Autodesk Inventor part; units mm, degrees
(part 2 of 3)
  arc A433 (-195.284, 57.8625) -> (-192.1375, 54.716) centre (-190, 60) ccw construction
  arc A434 (-198.1598, 81.4621) -> (-195.284, 57.8625) centre (-152.919, 75) ccw construction
  arc A435 (-196.5476, 84.6866) -> (-198.1598, 81.4621) centre (-192.5171, 80.6561) ccw construction
  line L149 (-196.5476, 84.6866) -> (-178.0824, 103.1518) construction
  arc A436 (-171.9305, 105.7) -> (-178.0824, 103.1518) centre (-171.9305, 97) ccw construction
  line L150 (-171.9305, 105.7) -> (-161.9122, 105.7) construction
  arc A437 (-192.1375, 45.284) -> (-195.284, 42.1375) centre (-190, 40) ccw construction
  arc A438 (-157.8625, 45.284) -> (-192.1375, 45.284) centre (-175, 2.919) ccw construction
  arc A439 (-154.716, 42.1375) -> (-157.8625, 45.284) centre (-160, 40) ccw construction
  arc A440 (-154.716, 7.8625) -> (-154.716, 42.1375) centre (-197.081, 25) ccw construction
  arc A441 (-157.8625, 4.716) -> (-154.716, 7.8625) centre (-160, 10) ccw construction
  arc A442 (-192.1375, 4.716) -> (-157.8625, 4.716) centre (-175, 47.081) ccw construction
  arc A443 (-195.284, 7.8625) -> (-192.1375, 4.716) centre (-190, 10) ccw construction
  arc A444 (-195.284, 42.1375) -> (-195.284, 7.8625) centre (-152.919, 25) ccw construction
  arc A445 (-192.1375, -4.716) -> (-195.284, -7.8625) centre (-190, -10) ccw construction
  arc A446 (-157.8625, -4.716) -> (-192.1375, -4.716) centre (-175, -47.081) ccw construction
  arc A447 (-154.716, -7.8625) -> (-157.8625, -4.716) centre (-160, -10) ccw construction
  arc A448 (-154.716, -42.1375) -> (-154.716, -7.8625) centre (-197.081, -25) ccw construction
  arc A449 (-157.8625, -45.284) -> (-154.716, -42.1375) centre (-160, -40) ccw construction
  arc A450 (-192.1375, -45.284) -> (-157.8625, -45.284) centre (-175, -2.919) ccw construction
  arc A451 (-195.284, -42.1375) -> (-192.1375, -45.284) centre (-190, -40) ccw construction
  arc A452 (-195.284, -7.8625) -> (-195.284, -42.1375) centre (-152.919, -25) ccw construction
  line L151 (-172.8179, -78.4527) -> (-172.8179, -89.3404) construction
  arc A453 (-183.0505, -97.9043) -> (-172.8179, -89.3404) centre (-181.5179, -89.3404) ccw construction
  arc A454 (-192.1375, -95.284) -> (-183.0505, -97.9043) centre (-175, -52.919) ccw construction
  arc A455 (-195.284, -92.1375) -> (-192.1375, -95.284) centre (-190, -90) ccw construction
  arc A456 (-195.284, -57.8625) -> (-195.284, -92.1375) centre (-152.919, -75) ccw construction
  arc A457 (-192.1375, -54.716) -> (-195.284, -57.8625) centre (-190, -60) ccw construction
  arc A458 (-171.3004, -51.531) -> (-192.1375, -54.716) centre (-175, -97.081) ccw construction
  arc A459 (-164.8787, -65.1933) -> (-171.3004, -51.531) centre (-172.0047, -60.2024) ccw construction
  line L152 (-164.8787, -65.1933) -> (-171.7143, -74.9534) construction
  arc A460 (-171.7143, -74.9534) -> (-172.8179, -78.4527) centre (-166.7179, -78.4527) ccw construction
  arc A461 (-195.284, -107.8625) -> (-198.5651, -122.7803) centre (-152.919, -125) ccw construction
  arc A462 (-192.1375, -104.716) -> (-195.284, -107.8625) centre (-190, -110) ccw construction
  arc A463 (-168.9997, -101.7766) -> (-192.1375, -104.716) centre (-175, -147.081) ccw construction
  arc A464 (-163.9859, -111.6056) -> (-168.9997, -101.7766) centre (-169.8794, -108.4186) ccw construction
  arc A465 (-163.9859, -111.6056) -> (-158.7814, -119.3988) centre (-159.3239, -114.1267) ccw construction
  arc A466 (-151.398, -126.2464) -> (-158.7814, -119.3988) centre (-158.0955, -126.0637) ccw construction
  arc A467 (-154.716, -142.1375) -> (-151.398, -126.2464) centre (-197.081, -125) ccw construction
  arc A468 (-157.8625, -145.284) -> (-154.716, -142.1375) centre (-160, -140) ccw construction
  arc A469 (-181.1757, -148.1998) -> (-157.8625, -145.284) centre (-175, -102.919) ccw construction
  arc A470 (-188.7, -139.5796) -> (-181.1757, -148.1998) centre (-180, -139.5796) ccw construction
  line L153 (-188.7, -139.5796) -> (-188.7, -137.0711) construction
  arc A471 (-188.7, -137.0711) -> (-189.9594, -134.0305) centre (-193, -137.0711) ccw construction
  line L154 (-189.9594, -134.0305) -> (-196.9023, -127.0876) construction
  arc A472 (-198.5651, -122.7803) -> (-196.9023, -127.0876) centre (-192.8718, -123.0571) ccw construction
  arc A473 (-157.8625, -154.716) -> (-171.7212, -151.4988) centre (-175, -197.081) ccw construction
  arc A474 (-154.716, -157.8625) -> (-157.8625, -154.716) centre (-160, -160) ccw construction
  arc A475 (-151.4988, -171.7212) -> (-154.716, -157.8625) centre (-197.081, -175) ccw construction
  arc A476 (-166.4392, -178.3841) -> (-151.4988, -171.7212) centre (-160.1763, -172.3454) ccw construction
  arc A477 (-166.4392, -178.3841) -> (-178.3841, -166.4392) centre (-500.278, -500.278) ccw construction
  arc A478 (-171.7212, -151.4988) -> (-178.3841, -166.4392) centre (-172.3454, -160.1763) ccw construction
  arc A479 (-107.8625, -195.284) -> (-104.716, -192.1375) centre (-110, -190) ccw construction
  arc A480 (-142.1375, -195.284) -> (-107.8625, -195.284) centre (-125, -152.919) ccw construction
  arc A481 (-145.284, -192.1375) -> (-142.1375, -195.284) centre (-140, -190) ccw construction
  arc A482 (-145.284, -157.8625) -> (-145.284, -192.1375) centre (-102.919, -175) ccw construction
  arc A483 (-142.1375, -154.716) -> (-145.284, -157.8625) centre (-140, -160) ccw construction
  arc A484 (-107.8625, -154.716) -> (-142.1375, -154.716) centre (-125, -197.081) ccw construction
  arc A485 (-104.716, -157.8625) -> (-107.8625, -154.716) centre (-110, -160) ccw construction
  arc A486 (-104.716, -192.1375) -> (-104.716, -157.8625) centre (-147.081, -175) ccw construction
  arc A487 (-128.4924, -148.4854) -> (-107.8625, -145.284) centre (-125, -102.919) ccw construction
  arc A488 (-133.4107, -144.758) -> (-128.4924, -148.4854) centre (-128.0568, -142.802) ccw construction
  arc A489 (-133.4107, -144.758) -> (-139.1817, -140.7513) centre (-139.1403, -146.8512) ccw construction
  arc A490 (-147.7814, -133.7096) -> (-139.1817, -140.7513) centre (-139.2409, -132.0515) ccw construction
  arc A491 (-145.284, -107.8625) -> (-147.7814, -133.7096) centre (-102.919, -125) ccw construction
  arc A492 (-142.1375, -104.716) -> (-145.284, -107.8625) centre (-140, -110) ccw construction
  arc A493 (-107.8625, -104.716) -> (-142.1375, -104.716) centre (-125, -147.081) ccw construction
  arc A494 (-104.716, -107.8625) -> (-107.8625, -104.716) centre (-110, -110) ccw construction
  arc A495 (-104.716, -142.1375) -> (-104.716, -107.8625) centre (-147.081, -125) ccw construction
  arc A496 (-107.8625, -145.284) -> (-104.716, -142.1375) centre (-110, -140) ccw construction
  arc A497 (-139.6902, -96.1936) -> (-142.6797, -95.7) centre (-142.6797, -105) ccw construction
  line L155 (-142.6797, -95.7) -> (-156, -95.7) construction
  arc A498 (-160.7, -91) -> (-156, -95.7) centre (-156, -91) ccw construction
  line L156 (-160.7, -91) -> (-160.7, -82.9939) construction
  arc A499 (-158.7642, -76.8556) -> (-160.7, -82.9939) centre (-150, -82.9939) ccw construction
  line L157 (-158.7642, -76.8556) -> (-144.6688, -56.7301) construction
  arc A500 (-142.1375, -54.716) -> (-144.6688, -56.7301) centre (-140, -60) ccw construction
  arc A501 (-107.8625, -54.716) -> (-142.1375, -54.716) centre (-125, -97.081) ccw construction
  arc A502 (-104.716, -57.8625) -> (-107.8625, -54.716) centre (-110, -60) ccw construction
  arc A503 (-104.716, -92.1375) -> (-104.716, -57.8625) centre (-147.081, -75) ccw construction
  arc A504 (-107.8625, -95.284) -> (-104.716, -92.1375) centre (-110, -90) ccw construction
  arc A505 (-139.6902, -96.1936) -> (-107.8625, -95.284) centre (-125, -52.919) ccw construction
  arc A506 (-142.1375, -4.716) -> (-145.284, -7.8625) centre (-140, -10) ccw construction
  arc A507 (-107.8625, -4.716) -> (-142.1375, -4.716) centre (-125, -47.081) ccw construction
  arc A508 (-104.716, -7.8625) -> (-107.8625, -4.716) centre (-110, -10) ccw construction
  arc A509 (-104.716, -42.1375) -> (-104.716, -7.8625) centre (-147.081, -25) ccw construction
  arc A510 (-107.8625, -45.284) -> (-104.716, -42.1375) centre (-110, -40) ccw construction
  arc A511 (-142.1375, -45.284) -> (-107.8625, -45.284) centre (-125, -2.919) ccw construction
  arc A512 (-145.284, -42.1375) -> (-142.1375, -45.284) centre (-140, -40) ccw construction
  arc A513 (-145.284, -7.8625) -> (-145.284, -42.1375) centre (-102.919, -25) ccw construction
  arc A514 (-92.1375, 45.284) -> (-95.284, 42.1375) centre (-90, 40) ccw construction
  arc A515 (-57.8625, 45.284) -> (-92.1375, 45.284) centre (-75, 2.919) ccw construction
  arc A516 (-54.716, 42.1375) -> (-57.8625, 45.284) centre (-60, 40) ccw projected
  arc A517 (-54.716, 7.8625) -> (-54.716, 42.1375) centre (-97.081, 25) ccw projected
  arc A518 (-57.8625, 4.716) -> (-54.716, 7.8625) centre (-60, 10) ccw projected
  arc A519 (-92.1375, 4.716) -> (-57.8625, 4.716) centre (-75, 47.081) ccw construction
  arc A520 (-95.284, 7.8625) -> (-92.1375, 4.716) centre (-90, 10) ccw construction
  arc A521 (-95.284, 42.1375) -> (-95.284, 7.8625) centre (-52.919, 25) ccw construction
  arc A522 (-45.3096, 30.6473) -> (-44.8166, 8.2343) centre (-7.9112, 20.258) ccw projected
  arc A523 (-29.5673, 37.0015) -> (-45.3096, 30.6473) centre (-35, 27.7833) ccw projected
  arc A524 (-29.5673, 37.0015) -> (-20.8305, 37.1926) centre (-25.3532, 44.1521) ccw projected
  arc A525 (-5.5366, 33.2142) -> (-20.8305, 37.1926) centre (-15, 28.2207) ccw projected
  arc A526 (-8.2916, 26.5347) -> (-5.5366, 33.2142) centre (-9.6934, 31.0208) ccw projected
  arc A527 (-8.2916, 26.5347) -> (-26.7128, 7.6985) centre (0, 0) ccw projected
  arc A528 (-31.229, 4.3) -> (-26.7128, 7.6985) centre (-31.229, 9) ccw projected
  line L158 (-31.229, 4.3) -> (-39.3969, 4.3) projected
  arc A529 (-44.8166, 8.2343) -> (-39.3969, 4.3) centre (-39.3969, 10) ccw projected
  arc A530 (-30.6473, -45.3096) -> (-8.2343, -44.8166) centre (-20.258, -7.9112) ccw projected
  arc A531 (-37.0015, -29.5673) -> (-30.6473, -45.3096) centre (-27.7833, -35) ccw projected
  arc A532 (-37.0015, -29.5673) -> (-37.1926, -20.8305) centre (-44.1521, -25.3532) ccw projected
  arc A533 (-33.2142, -5.5366) -> (-37.1926, -20.8305) centre (-28.2207, -15) ccw projected
  arc A534 (-26.5347, -8.2916) -> (-33.2142, -5.5366) centre (-31.0208, -9.6934) ccw projected
  arc A535 (-26.5347, -8.2916) -> (-7.6985, -26.7128) centre (0, 0) ccw projected
  arc A536 (-4.3, -31.229) -> (-7.6985, -26.7128) centre (-9, -31.229) ccw projected
  line L159 (-4.3, -31.229) -> (-4.3, -39.3969) projected
  arc A537 (-8.2343, -44.8166) -> (-4.3, -39.3969) centre (-10, -39.3969) ccw projected
  arc A538 (-92.1375, -4.716) -> (-95.284, -7.8625) centre (-90, -10) ccw construction
  arc A539 (-57.8625, -4.716) -> (-92.1375, -4.716) centre (-75, -47.081) ccw construction
  arc A540 (-54.716, -7.8625) -> (-57.8625, -4.716) centre (-60, -10) ccw projected
  arc A541 (-54.716, -42.1375) -> (-54.716, -7.8625) centre (-97.081, -25) ccw projected
  arc A542 (-57.8625, -45.284) -> (-54.716, -42.1375) centre (-60, -40) ccw projected
  arc A543 (-92.1375, -45.284) -> (-57.8625, -45.284) centre (-75, -2.919) ccw construction
  arc A544 (-95.284, -42.1375) -> (-92.1375, -45.284) centre (-90, -40) ccw construction
  arc A545 (-95.284, -7.8625) -> (-95.284, -42.1375) centre (-52.919, -25) ccw construction
  arc A546 (-92.1375, -54.716) -> (-95.284, -57.8625) centre (-90, -60) ccw construction
  arc A547 (-57.8625, -54.716) -> (-92.1375, -54.716) centre (-75, -97.081) ccw construction
  arc A548 (-54.716, -57.8625) -> (-57.8625, -54.716) centre (-60, -60) ccw projected
  arc A549 (-54.716, -92.1375) -> (-54.716, -57.8625) centre (-97.081, -75) ccw construction
  arc A550 (-57.8625, -95.284) -> (-54.716, -92.1375) centre (-60, -90) ccw construction
  arc A551 (-92.1375, -95.284) -> (-57.8625, -95.284) centre (-75, -52.919) ccw construction
  arc A552 (-95.284, -92.1375) -> (-92.1375, -95.284) centre (-90, -90) ccw construction
  arc A553 (-95.284, -57.8625) -> (-95.284, -92.1375) centre (-52.919, -75) ccw construction
  arc A554 (-92.1375, -104.716) -> (-95.284, -107.8625) centre (-90, -110) ccw construction
  arc A555 (-57.8625, -104.716) -> (-92.1375, -104.716) centre (-75, -147.081) ccw construction
  arc A556 (-54.716, -107.8625) -> (-57.8625, -104.716) centre (-60, -110) ccw construction
  arc A557 (-54.716, -142.1375) -> (-54.716, -107.8625) centre (-97.081, -125) ccw construction
  arc A558 (-57.8625, -145.284) -> (-54.716, -142.1375) centre (-60, -140) ccw construction
  arc A559 (-92.1375, -145.284) -> (-57.8625, -145.284) centre (-75, -102.919) ccw construction
  arc A560 (-95.284, -142.1375) -> (-92.1375, -145.284) centre (-90, -140) ccw construction
  arc A561 (-95.284, -107.8625) -> (-95.284, -142.1375) centre (-52.919, -125) ccw construction
  arc A562 (-92.1375, -154.716) -> (-95.284, -157.8625) centre (-90, -160) ccw construction
  arc A563 (-57.8625, -154.716) -> (-92.1375, -154.716) centre (-75, -197.081) ccw construction
  arc A564 (-54.716, -157.8625) -> (-57.8625, -154.716) centre (-60, -160) ccw construction
  arc A565 (-54.716, -192.1375) -> (-54.716, -157.8625) centre (-97.081, -175) ccw construction
  arc A566 (-57.8625, -195.284) -> (-54.716, -192.1375) centre (-60, -190) ccw construction
  arc A567 (-92.1375, -195.284) -> (-57.8625, -195.284) centre (-75, -152.919) ccw construction
  arc A568 (-95.284, -192.1375) -> (-92.1375, -195.284) centre (-90, -190) ccw construction
  arc A569 (-95.284, -157.8625) -> (-95.284, -192.1375) centre (-52.919, -175) ccw construction
  arc A570 (30.6473, 45.3096) -> (8.2343, 44.8166) centre (20.258, 7.9112) ccw projected
  arc A571 (37.0015, 29.5673) -> (30.6473, 45.3096) centre (27.7833, 35) ccw projected
  arc A572 (37.0015, 29.5673) -> (37.1926, 20.8305) centre (44.1521, 25.3532) ccw projected
  arc A573 (33.2142, 5.5366) -> (37.1926, 20.8305) centre (28.2207, 15) ccw projected
  arc A574 (26.5347, 8.2916) -> (33.2142, 5.5366) centre (31.0208, 9.6934) ccw projected
  arc A575 (26.5347, 8.2916) -> (7.6985, 26.7128) centre (0, 0) ccw projected
  arc A576 (4.3, 31.229) -> (7.6985, 26.7128) centre (9, 31.229) ccw projected
  line L160 (4.3, 31.229) -> (4.3, 39.3969) projected
  arc A577 (8.2343, 44.8166) -> (4.3, 39.3969) centre (10, 39.3969) ccw projected
  arc A578 (8.2916, -26.5347) -> (5.5366, -33.2142) centre (9.6934, -31.0208) ccw projected
  arc A579 (8.2916, -26.5347) -> (26.7128, -7.6985) centre (0, 0) ccw projected
  arc A580 (31.229, -4.3) -> (26.7128, -7.6985) centre (31.229, -9) ccw projected
  line L161 (31.229, -4.3) -> (39.3969, -4.3) projected
  arc A581 (44.8166, -8.2343) -> (39.3969, -4.3) centre (39.3969, -10) ccw projected
  arc A582 (45.3096, -30.6473) -> (44.8166, -8.2343) centre (7.9112, -20.258) ccw projected
  arc A583 (29.5673, -37.0015) -> (45.3096, -30.6473) centre (35, -27.7833) ccw projected
  arc A584 (29.5673, -37.0015) -> (20.8305, -37.1926) centre (25.3532, -44.1521) ccw projected
  arc A585 (5.5366, -33.2142) -> (20.8305, -37.1926) centre (15, -28.2207) ccw projected
  arc A586 (57.8625, 45.284) -> (54.716, 42.1375) centre (60, 40) ccw projected
  arc A587 (92.1375, 45.284) -> (57.8625, 45.284) centre (75, 2.919) ccw construction
  arc A588 (95.284, 42.1375) -> (92.1375, 45.284) centre (90, 40) ccw construction
  arc A589 (95.284, 7.8625) -> (95.284, 42.1375) centre (52.919, 25) ccw construction
  arc A590 (92.1375, 4.716) -> (95.284, 7.8625) centre (90, 10) ccw construction
  arc A591 (57.8625, 4.716) -> (92.1375, 4.716) centre (75, 47.081) ccw construction
  arc A592 (54.716, 7.8625) -> (57.8625, 4.716) centre (60, 10) ccw projected
  arc A593 (54.716, 42.1375) -> (54.716, 7.8625) centre (97.081, 25) ccw projected
  arc A594 (57.8625, -4.716) -> (54.716, -7.8625) centre (60, -10) ccw projected
  arc A595 (92.1375, -4.716) -> (57.8625, -4.716) centre (75, -47.081) ccw construction
  arc A596 (95.284, -7.8625) -> (92.1375, -4.716) centre (90, -10) ccw construction
  arc A597 (95.284, -42.1375) -> (95.284, -7.8625) centre (52.919, -25) ccw construction
  arc A598 (92.1375, -45.284) -> (95.284, -42.1375) centre (90, -40) ccw construction
  arc A599 (57.8625, -45.284) -> (92.1375, -45.284) centre (75, -2.919) ccw construction
  arc A600 (54.716, -42.1375) -> (57.8625, -45.284) centre (60, -40) ccw projected
  arc A601 (54.716, -7.8625) -> (54.716, -42.1375) centre (97.081, -25) ccw projected
  arc A602 (157.8625, 45.284) -> (154.716, 42.1375) centre (160, 40) ccw construction
  arc A603 (192.1375, 45.284) -> (157.8625, 45.284) centre (175, 2.919) ccw construction
  arc A604 (195.284, 42.1375) -> (192.1375, 45.284) centre (190, 40) ccw construction
  arc A605 (195.284, 7.8625) -> (195.284, 42.1375) centre (152.919, 25) ccw construction
  arc A606 (192.1375, 4.716) -> (195.284, 7.8625) centre (190, 10) ccw construction
  arc A607 (157.8625, 4.716) -> (192.1375, 4.716) centre (175, 47.081) ccw construction
  arc A608 (154.716, 7.8625) -> (157.8625, 4.716) centre (160, 10) ccw construction
  arc A609 (154.716, 42.1375) -> (154.716, 7.8625) centre (197.081, 25) ccw construction
  arc A610 (107.8625, 45.284) -> (104.716, 42.1375) centre (110, 40) ccw construction
  arc A611 (142.1375, 45.284) -> (107.8625, 45.284) centre (125, 2.919) ccw construction
  arc A612 (145.284, 42.1375) -> (142.1375, 45.284) centre (140, 40) ccw construction
  arc A613 (145.284, 7.8625) -> (145.284, 42.1375) centre (102.919, 25) ccw construction
  arc A614 (142.1375, 4.716) -> (145.284, 7.8625) centre (140, 10) ccw construction
  arc A615 (107.8625, 4.716) -> (142.1375, 4.716) centre (125, 47.081) ccw construction
  arc A616 (104.716, 7.8625) -> (107.8625, 4.716) centre (110, 10) ccw construction
  arc A617 (104.716, 42.1375) -> (104.716, 7.8625) centre (147.081, 25) ccw construction
  arc A618 (107.8625, -4.716) -> (104.716, -7.8625) centre (110, -10) ccw construction
  arc A619 (142.1375, -4.716) -> (107.8625, -4.716) centre (125, -47.081) ccw construction
  arc A620 (145.284, -7.8625) -> (142.1375, -4.716) centre (140, -10) ccw construction
  arc A621 (145.284, -42.1375) -> (145.284, -7.8625) centre (102.919, -25) ccw construction
  arc A622 (142.1375, -45.284) -> (145.284, -42.1375) centre (140, -40) ccw construction
  arc A623 (107.8625, -45.284) -> (142.1375, -45.284) centre (125, -2.919) ccw construction
  arc A624 (104.716, -42.1375) -> (107.8625, -45.284) centre (110, -40) ccw construction
  arc A625 (104.716, -7.8625) -> (104.716, -42.1375) centre (147.081, -25) ccw construction
  arc A626 (157.8625, -4.716) -> (154.716, -7.8625) centre (160, -10) ccw construction
  arc A627 (192.1375, -4.716) -> (157.8625, -4.716) centre (175, -47.081) ccw construction
  arc A628 (195.284, -7.8625) -> (192.1375, -4.716) centre (190, -10) ccw construction
  arc A629 (195.284, -42.1375) -> (195.284, -7.8625) centre (152.919, -25) ccw construction
  arc A630 (192.1375, -45.284) -> (195.284, -42.1375) centre (190, -40) ccw construction
  arc A631 (157.8625, -45.284) -> (192.1375, -45.284) centre (175, -2.919) ccw construction
  arc A632 (154.716, -42.1375) -> (157.8625, -45.284) centre (160, -40) ccw construction
  arc A633 (154.716, -7.8625) -> (154.716, -42.1375) centre (197.081, -25) ccw construction
  line L162 (157.3723, -102.2164) -> (154.5817, -91.8019) construction
  arc A634 (154.716, -57.8625) -> (154.5817, -91.8019) centre (197.081, -75) ccw construction
  arc A635 (157.8625, -54.716) -> (154.716, -57.8625) centre (160, -60) ccw construction
  arc A636 (192.1375, -54.716) -> (157.8625, -54.716) centre (175, -97.081) ccw construction
  arc A637 (195.284, -57.8625) -> (192.1375, -54.716) centre (190, -60) ccw construction
  arc A638 (198.1598, -81.4621) -> (195.284, -57.8625) centre (152.919, -75) ccw construction
  arc A639 (196.5476, -84.6866) -> (198.1598, -81.4621) centre (192.5171, -80.6561) ccw construction
  line L163 (196.5476, -84.6866) -> (178.0824, -103.1518) construction
  arc A640 (171.9305, -105.7) -> (178.0824, -103.1518) centre (171.9305, -97) ccw construction
  line L164 (171.9305, -105.7) -> (161.9122, -105.7) construction
  arc A641 (157.3723, -102.2164) -> (161.9122, -105.7) centre (161.9122, -101) ccw construction
  arc A642 (188.629, -104.3) -> (184.5985, -105.9695) centre (188.629, -110) ccw construction
  line L165 (188.629, -104.3) -> (190, -104.3) construction
  arc A643 (195.284, -107.8625) -> (190, -104.3) centre (190, -110) ccw construction
  arc A644 (198.5651, -122.7803) -> (195.284, -107.8625) centre (152.919, -125) ccw construction
  arc A645 (196.9023, -127.0876) -> (198.5651, -122.7803) centre (192.8718, -123.0571) ccw construction
  line L166 (196.9023, -127.0876) -> (189.9594, -134.0305) construction
  arc A646 (189.9594, -134.0305) -> (188.7, -137.0711) centre (193, -137.0711) ccw construction
  line L167 (188.7, -137.0711) -> (188.7, -139.5796) construction
  arc A647 (181.1757, -148.1998) -> (188.7, -139.5796) centre (180, -139.5796) ccw construction
  arc A648 (157.8625, -145.284) -> (181.1757, -148.1998) centre (175, -102.919) ccw construction
  arc A649 (154.716, -142.1375) -> (157.8625, -145.284) centre (160, -140) ccw construction
  arc A650 (151.6379, -129.8385) -> (154.716, -142.1375) centre (197.081, -125) ccw construction
  arc A651 (160.289, -120.2174) -> (151.6379, -129.8385) centre (160.289, -128.9174) ccw construction
  line L168 (160.289, -120.2174) -> (167.8239, -120.2174) construction
  arc A652 (167.8239, -120.2174) -> (172.1372, -118.4308) centre (167.8239, -114.1174) ccw construction
  line L169 (172.1372, -118.4308) -> (184.5985, -105.9695) construction
  arc A653 (195.3029, -159.9476) -> (191.4845, -156.1292) centre (193.3937, -158.0384) ccw construction
  line L170 (195.3029, -159.9476) -> (159.9476, -195.3029) construction
  arc A654 (156.1292, -191.4845) -> (159.9476, -195.3029) centre (158.0384, -193.3937) ccw construction
  line L171 (156.1292, -191.4845) -> (191.4845, -156.1292) construction
  arc A655 (154.716, -157.8625) -> (151.4988, -171.7212) centre (197.081, -175) ccw construction
  arc A656 (157.8625, -154.716) -> (154.716, -157.8625) centre (160, -160) ccw construction
  arc A657 (171.7212, -151.4988) -> (157.8625, -154.716) centre (175, -197.081) ccw construction
  arc A658 (178.3841, -166.4392) -> (171.7212, -151.4988) centre (172.3454, -160.1763) ccw construction
  arc A659 (178.3841, -166.4392) -> (166.4392, -178.3841) centre (500.278, -500.278) ccw construction
  arc A660 (151.4988, -171.7212) -> (166.4392, -178.3841) centre (160.1763, -172.3454) ccw construction
  arc A661 (-42.1375, -54.716) -> (-45.284, -57.8625) centre (-40, -60) ccw projected
  arc A662 (-7.8625, -54.716) -> (-42.1375, -54.716) centre (-25, -97.081) ccw projected
  arc A663 (-4.716, -57.8625) -> (-7.8625, -54.716) centre (-10, -60) ccw projected
  arc A664 (-4.716, -92.1375) -> (-4.716, -57.8625) centre (-47.081, -75) ccw construction
  arc A665 (-7.8625, -95.284) -> (-4.716, -92.1375) centre (-10, -90) ccw construction
  arc A666 (-42.1375, -95.284) -> (-7.8625, -95.284) centre (-25, -52.919) ccw construction
  arc A667 (-45.284, -92.1375) -> (-42.1375, -95.284) centre (-40, -90) ccw construction
  arc A668 (-45.284, -57.8625) -> (-45.284, -92.1375) centre (-2.919, -75) ccw construction
  arc A669 (7.8625, -54.716) -> (4.716, -57.8625) centre (10, -60) ccw projected
  arc A670 (42.1375, -54.716) -> (7.8625, -54.716) centre (25, -97.081) ccw projected
  arc A671 (45.284, -57.8625) -> (42.1375, -54.716) centre (40, -60) ccw projected
  arc A672 (45.284, -92.1375) -> (45.284, -57.8625) centre (2.919, -75) ccw construction
  arc A673 (42.1375, -95.284) -> (45.284, -92.1375) centre (40, -90) ccw construction
  arc A674 (7.8625, -95.284) -> (42.1375, -95.284) centre (25, -52.919) ccw construction
  arc A675 (4.716, -92.1375) -> (7.8625, -95.284) centre (10, -90) ccw construction
  arc A676 (4.716, -57.8625) -> (4.716, -92.1375) centre (47.081, -75) ccw construction
  arc A677 (57.8625, -54.716) -> (54.716, -57.8625) centre (60, -60) ccw projected
  arc A678 (92.1375, -54.716) -> (57.8625, -54.716) centre (75, -97.081) ccw construction
  arc A679 (95.284, -57.8625) -> (92.1375, -54.716) centre (90, -60) ccw construction
  arc A680 (95.284, -92.1375) -> (95.284, -57.8625) centre (52.919, -75) ccw construction
  arc A681 (92.1375, -95.284) -> (95.284, -92.1375) centre (90, -90) ccw construction
  arc A682 (57.8625, -95.284) -> (92.1375, -95.284) centre (75, -52.919) ccw construction
  arc A683 (54.716, -92.1375) -> (57.8625, -95.284) centre (60, -90) ccw construction
  arc A684 (54.716, -57.8625) -> (54.716, -92.1375) centre (97.081, -75) ccw construction
  arc A685 (107.8625, -54.716) -> (104.716, -57.8625) centre (110, -60) ccw construction
  arc A686 (142.1375, -54.716) -> (107.8625, -54.716) centre (125, -97.081) ccw construction
  arc A687 (145.284, -57.8625) -> (142.1375, -54.716) centre (140, -60) ccw construction
  arc A688 (145.284, -92.1375) -> (145.284, -57.8625) centre (102.919, -75) ccw construction
  arc A689 (142.1375, -95.284) -> (145.284, -92.1375) centre (140, -90) ccw construction
  arc A690 (107.8625, -95.284) -> (142.1375, -95.284) centre (125, -52.919) ccw construction
  arc A691 (104.716, -92.1375) -> (107.8625, -95.284) centre (110, -90) ccw construction
  arc A692 (104.716, -57.8625) -> (104.716, -92.1375) centre (147.081, -75) ccw construction
  arc A693 (107.8625, -104.716) -> (104.716, -107.8625) centre (110, -110) ccw construction
  arc A694 (142.1375, -104.716) -> (107.8625, -104.716) centre (125, -147.081) ccw construction
  arc A695 (145.284, -107.8625) -> (142.1375, -104.716) centre (140, -110) ccw construction
  arc A696 (145.284, -142.1375) -> (145.284, -107.8625) centre (102.919, -125) ccw construction
  arc A697 (142.1375, -145.284) -> (145.284, -142.1375) centre (140, -140) ccw construction
  arc A698 (107.8625, -145.284) -> (142.1375, -145.284) centre (125, -102.919) ccw construction
  arc A699 (104.716, -142.1375) -> (107.8625, -145.284) centre (110, -140) ccw construction
  arc A700 (104.716, -107.8625) -> (104.716, -142.1375) centre (147.081, -125) ccw construction
  arc A701 (95.284, -107.8625) -> (92.1375, -104.716) centre (90, -110) ccw construction
  arc A702 (96.1936, -139.6902) -> (95.284, -107.8625) centre (52.919, -125) ccw construction
  arc A703 (96.1936, -139.6902) -> (95.7, -142.6797) centre (105, -142.6797) ccw construction
  line L172 (95.7, -142.6797) -> (95.7, -156) construction
  arc A704 (91, -160.7) -> (95.7, -156) centre (91, -156) ccw construction
  line L173 (91, -160.7) -> (82.9939, -160.7) construction
  arc A705 (76.8556, -158.7642) -> (82.9939, -160.7) centre (82.9939, -150) ccw construction
  line L174 (76.8556, -158.7642) -> (56.7301, -144.6688) construction
  arc A706 (54.716, -142.1375) -> (56.7301, -144.6688) centre (60, -140) ccw construction
  arc A707 (54.716, -107.8625) -> (54.716, -142.1375) centre (97.081, -125) ccw construction
  arc A708 (57.8625, -104.716) -> (54.716, -107.8625) centre (60, -110) ccw construction
  arc A709 (92.1375, -104.716) -> (57.8625, -104.716) centre (75, -147.081) ccw construction
  arc A710 (7.8625, -104.716) -> (4.716, -107.8625) centre (10, -110) ccw construction
  arc A711 (42.1375, -104.716) -> (7.8625, -104.716) centre (25, -147.081) ccw construction
  arc A712 (45.284, -107.8625) -> (42.1375, -104.716) centre (40, -110) ccw construction
  arc A713 (45.284, -142.1375) -> (45.284, -107.8625) centre (2.919, -125) ccw construction
  arc A714 (42.1375, -145.284) -> (45.284, -142.1375) centre (40, -140) ccw construction
  arc A715 (7.8625, -145.284) -> (42.1375, -145.284) centre (25, -102.919) ccw construction
  arc A716 (4.716, -142.1375) -> (7.8625, -145.284) centre (10, -140) ccw construction
  arc A717 (4.716, -107.8625) -> (4.716, -142.1375) centre (47.081, -125) ccw construction
  arc A718 (-42.1375, -104.716) -> (-45.284, -107.8625) centre (-40, -110) ccw construction
  arc A719 (-7.8625, -104.716) -> (-42.1375, -104.716) centre (-25, -147.081) ccw construction
  arc A720 (-4.716, -107.8625) -> (-7.8625, -104.716) centre (-10, -110) ccw construction
  arc A721 (-4.716, -142.1375) -> (-4.716, -107.8625) centre (-47.081, -125) ccw construction
  arc A722 (-7.8625, -145.284) -> (-4.716, -142.1375) centre (-10, -140) ccw construction
  arc A723 (-42.1375, -145.284) -> (-7.8625, -145.284) centre (-25, -102.919) ccw construction
  arc A724 (-45.284, -142.1375) -> (-42.1375, -145.284) centre (-40, -140) ccw construction
  arc A725 (-45.284, -107.8625) -> (-45.284, -142.1375) centre (-2.919, -125) ccw construction
  arc A726 (-4.7057, -157.8881) -> (-7.8625, -154.716) centre (-10, -160) ccw construction
  spline S4 degree 3 poles (-4.7061, -157.8883) (-4.2708, -159.1004) (-3.9515, -160.1229) (-3.8345, -161.8168) (-3.8428, -162.3944) (-3.9938, -163.7605) (-4.0841, -164.1049) (-4.2294, -164.796) knots -0.869704 -0.869704 -0.869704 -0.869704 -0.412328 -0.412328 -0.211846 -0.211846 0 0 0 0 construction
  arc A727 (-4.2294, -164.796) -> (-4.3, -165.4748) centre (-1, -165.4748) ccw construction
  line L175 (-4.3, -165.4748) -> (-4.3, -180.5) construction
  arc A728 (-4.3, -180.5) -> (-4.2569, -181.1076) centre (0, -180.5) ccw construction
  arc A729 (-7.9197, -185.3304) -> (-4.2569, -181.1076) centre (-7.9197, -181.6304) ccw construction
  line L176 (-7.9197, -185.3304) -> (-29.7064, -185.3304) construction
  arc A730 (-29.7064, -185.3304) -> (-34.5086, -186.9839) centre (-29.7064, -193.1304) ccw construction
  line L177 (-34.5086, -186.9839) -> (-37.4772, -189.3032) construction
  arc A731 (-37.4772, -189.3032) -> (-39.2734, -191.2903) centre (-32.675, -195.4497) ccw construction
  arc A732 (-45.8818, -190.5785) -> (-39.2734, -191.2903) centre (-42.4034, -189.3172) ccw construction
  arc A733 (-45.284, -157.8625) -> (-45.8818, -190.5785) centre (-2.919, -175) ccw construction
  arc A734 (-42.1375, -154.716) -> (-45.284, -157.8625) centre (-40, -160) ccw construction
  arc A735 (-7.8625, -154.716) -> (-42.1375, -154.716) centre (-25, -197.081) ccw construction
  arc A736 (4.3, -165.4748) -> (4.2294, -164.796) centre (1, -165.4748) ccw construction
  spline S5 degree 3 poles (4.2294, -164.796) (4.0839, -164.1041) (3.9936, -163.7593) (3.8433, -162.3972) (3.8343, -161.82) (3.9511, -160.1263) (4.265, -159.1168) (4.7061, -157.8883) knots -0.748459 -0.748459 -0.748459 -0.748459 -0.564349 -0.564349 -0.391594 -0.391594 0 0 0 0 construction
  arc A737 (7.8625, -154.716) -> (4.7057, -157.8881) centre (10, -160) ccw construction
  arc A738 (42.1375, -154.716) -> (7.8625, -154.716) centre (25, -197.081) ccw construction
  arc A739 (45.284, -157.8625) -> (42.1375, -154.716) centre (40, -160) ccw construction
  arc A740 (45.8818, -190.5785) -> (45.284, -157.8625) centre (2.919, -175) ccw construction
  arc A741 (39.2734, -191.2903) -> (45.8818, -190.5785) centre (42.4034, -189.3172) ccw construction
  arc A742 (39.2734, -191.2903) -> (37.4772, -189.3032) centre (32.675, -195.4497) ccw construction
  line L178 (37.4772, -189.3032) -> (34.5086, -186.9839) construction
  arc A743 (34.5086, -186.9839) -> (29.7064, -185.3304) centre (29.7064, -193.1304) ccw construction
  line L179 (29.7064, -185.3304) -> (7.9197, -185.3304) construction
  arc A744 (4.2569, -181.1076) -> (7.9197, -185.3304) centre (7.9197, -181.6304) ccw construction
  arc A745 (4.2569, -181.1076) -> (4.3, -180.5) centre (0, -180.5) ccw construction
  line L180 (4.3, -180.5) -> (4.3, -165.4748) construction
  line L181 (65.1933, -164.8787) -> (74.9534, -171.7143) construction
  arc A746 (74.9534, -171.7143) -> (78.4527, -172.8179) centre (78.4527, -166.7179) ccw construction
  line L182 (78.4527, -172.8179) -> (89.3404, -172.8179) construction
  arc A747 (97.9043, -183.0505) -> (89.3404, -172.8179) centre (89.3404, -181.5179) ccw construction
  arc A748 (95.284, -192.1375) -> (97.9043, -183.0505) centre (52.919, -175) ccw construction
  arc A749 (92.1375, -195.284) -> (95.284, -192.1375) centre (90, -190) ccw construction
  arc A750 (57.8625, -195.284) -> (92.1375, -195.284) centre (75, -152.919) ccw construction
  arc A751 (54.716, -192.1375) -> (57.8625, -195.284) centre (60, -190) ccw construction
  arc A752 (51.531, -171.3004) -> (54.716, -192.1375) centre (97.081, -175) ccw construction
  arc A753 (65.1933, -164.8787) -> (51.531, -171.3004) centre (60.2024, -172.0047) ccw construction
  arc A754 (104.716, -192.1375) -> (107.8625, -195.284) centre (110, -190) ccw construction
  arc A755 (104.716, -157.8625) -> (104.716, -192.1375) centre (147.081, -175) ccw construction
  arc A756 (107.8625, -154.716) -> (104.716, -157.8625) centre (110, -160) ccw construction
  arc A757 (142.1375, -154.716) -> (107.8625, -154.716) centre (125, -197.081) ccw construction
  arc A758 (145.284, -157.8625) -> (142.1375, -154.716) centre (140, -160) ccw construction
  arc A759 (145.284, -192.1375) -> (145.284, -157.8625) centre (102.919, -175) ccw construction
  arc A760 (142.1375, -195.284) -> (145.284, -192.1375) centre (140, -190) ccw construction
  arc A761 (107.8625, -195.284) -> (142.1375, -195.284) centre (125, -152.919) ccw construction
  circle A762 centre (159.3239, 114.1267) radius 3.36 construction
  circle A763 centre (-159.3239, -114.1267) radius 3.36 construction
  circle A764 centre (0, -180.5) radius 3.36 construction
  circle A765 centre (0, -164.5) radius 3.36 construction
  circle A766 centre (0, 164.5) radius 3.36 construction
  circle A767 centre (0, 180.5) radius 3.36 construction
  circle A768 centre (160.3736, 69.3944) radius 3.36 construction
  circle A769 centre (166.7179, 78.4527) radius 3.36 construction
  circle A770 centre (139.1403, 146.8512) radius 3.36 construction
  circle A771 centre (-69.3944, 160.3736) radius 3.36 construction
  circle A772 centre (-78.4527, 166.7179) radius 3.36 construction
  circle A773 centre (-159.3239, 114.1267) radius 3.36 construction
  circle A774 centre (-167.8239, 114.1174) radius 3.36 construction
  circle A775 centre (-166.7179, -78.4527) radius 3.36 construction
  circle A776 centre (-160.3736, -69.3944) radius 3.36 construction
  circle A777 centre (-139.1403, -146.8512) radius 3.36 construction
  circle A778 centre (159.3239, -114.1267) radius 3.36 construction
  circle A779 centre (167.8239, -114.1174) radius 3.36 construction
  circle A780 centre (69.3944, -160.3736) radius 3.36 construction
  circle A781 centre (78.4527, -166.7179) radius 3.36 construction
  circle A782 centre (-193.6137, 137.7365) radius 3.36 construction
  circle A783 centre (-201.6137, 137.7365) radius 3.36 construction
  circle A784 centre (-193.6137, -137.7365) radius 3.36 construction
  circle A785 centre (-201.6137, -137.7365) radius 3.36 construction
  circle A786 centre (193.6137, 137.7365) radius 3.36 construction
  circle A787 centre (201.6137, 137.7365) radius 3.36 construction
  circle A788 centre (193.6137, -137.7365) radius 3.36 construction
  circle A789 centre (201.6137, -137.7365) radius 3.36 construction
  circle A790 centre (150, -150) radius 2.15 construction
  circle A791 centre (150, -100) radius 2.15 construction
  circle A792 centre (150, -50) radius 2.15 construction
  circle A793 centre (150, 0) radius 2.15 construction
  circle A794 centre (150, 50) radius 2.15 construction
  circle A795 centre (150, 100) radius 2.15 construction
  circle A796 centre (150, 150) radius 2.15 construction
  circle A797 centre (-150, -150) radius 2.15 construction
  circle A798 centre (-100, -150) radius 2.15 construction
  circle A799 centre (-50, -150) radius 2.15 construction
  circle A800 centre (0, -150) radius 2.15 construction
  circle A801 centre (50, -150) radius 2.15 construction
  circle A802 centre (100, -150) radius 2.15 construction
  circle A803 centre (-150, -100) radius 2.15 construction
  circle A804 centre (-100, -100) radius 2.15 construction
  circle A805 centre (-50, -100) radius 2.15 construction
  circle A806 centre (0, -100) radius 2.15 construction
  circle A807 centre (50, -100) radius 2.15 construction
  circle A808 centre (100, -100) radius 2.15 construction
  circle A809 centre (-150, -50) radius 2.15 construction
  circle A810 centre (-100, -50) radius 2.15 construction
  circle A811 centre (-50, -50) radius 2.15 construction
  circle A812 centre (0, -50) radius 2.15 construction
  circle A813 centre (50, -50) radius 2.15 construction
  circle A814 centre (100, -50) radius 2.15 construction
  circle A815 centre (-150, 0) radius 2.15 construction
  circle A816 centre (-100, 0) radius 2.15 construction
  circle A817 centre (-50, 0) radius 2.15 construction
  circle A818 centre (50, 0) radius 2.15 construction
  circle A819 centre (100, 0) radius 2.15 construction
  circle A820 centre (-150, 50) radius 2.15 construction
  circle A821 centre (-100, 50) radius 2.15 construction
  circle A822 centre (-50, 50) radius 2.15 construction
  circle A823 centre (0, 50) radius 2.15 construction
  circle A824 centre (50, 50) radius 2.15 construction
  circle A825 centre (100, 50) radius 2.15 construction
  circle A826 centre (-150, 100) radius 2.15 construction
  circle A827 centre (-100, 100) radius 2.15 construction
  circle A828 centre (-50, 100) radius 2.15 construction
  circle A829 centre (0, 100) radius 2.15 construction
  circle A830 centre (50, 100) radius 2.15 construction
  circle A831 centre (100, 100) radius 2.15 construction
  circle A832 centre (-50, 150) radius 2.15 construction
  circle A833 centre (0, 150) radius 2.15 construction
  circle A834 centre (50, 150) radius 2.15 construction
  circle A835 centre (100, 150) radius 2.15 construction
  circle A836 centre (44.1521, 25.3532) radius 4.48 construction
  circle A837 centre (-25.3532, 44.1521) radius 4.48 construction
  circle A838 centre (-44.1521, -25.3532) radius 4.48 projected
  circle A839 centre (25.3532, -44.1521) radius 4.48 construction
  circle A840 centre (-22.6274, 0) radius 4.48 projected
  circle A841 centre (0, 22.6274) radius 4.48 projected
  circle A842 centre (22.6274, 0) radius 4.48 projected
  circle A843 centre (0, -22.6274) radius 4.48 projected
  circle A844 centre (16, 16) radius 2.4 projected
  circle A845 centre (16, -16) radius 2.4 projected
  circle A846 centre (-16, 16) radius 2.4 projected
  circle A847 centre (-16, -16) radius 2.4 projected
  circle A848 centre (20.2008, -8.7138) radius 3.15 projected
  circle A849 centre (-20.2008, 8.7138) radius 3.15 projected
  arc A850 (-148.6506, 142.3094) -> (-150.5101, 138.3216) centre (-149.5803, 140.3155) ccw construction
  arc A851 (-148.6506, 142.3094) -> (-104.0109, 162.4745) centre (-135, 171.5831) ccw construction
  arc A852 (-99.7895, 161.2337) -> (-104.0109, 162.4745) centre (-101.9002, 161.8541) ccw construction
  arc A853 (-150.5101, 138.3216) -> (-99.7895, 161.2337) centre (-135, 171.5831) ccw construction
  arc A854 (204.5, -108.5) -> (200.1, -108.5) centre (202.3, -108.5) ccw construction
  line L183 (204.5, -108.5) -> (204.5, -128.5) construction
  arc A855 (200.1, -128.5) -> (204.5, -128.5) centre (202.3, -128.5) ccw construction
  line L184 (200.1, -128.5) -> (200.1, -108.5) construction
  arc A856 (204.5, -65) -> (200.1, -65) centre (202.3, -65) ccw construction
  line L185 (204.5, -65) -> (204.5, -85) construction
  arc A857 (200.1, -85) -> (204.5, -85) centre (202.3, -85) ccw construction
  line L186 (200.1, -85) -> (200.1, -65) construction
  arc A858 (204.5, -15) -> (200.1, -15) centre (202.3, -15) ccw construction
  line L187 (204.5, -15) -> (204.5, -35) construction
  arc A859 (200.1, -35) -> (204.5, -35) centre (202.3, -35) ccw construction
  line L188 (200.1, -35) -> (200.1, -15) construction
  arc A860 (204.5, 35) -> (200.1, 35) centre (202.3, 35) ccw construction
  line L189 (204.5, 35) -> (204.5, 15) construction
  arc A861 (200.1, 15) -> (204.5, 15) centre (202.3, 15) ccw construction
  line L190 (200.1, 15) -> (200.1, 35) construction
  arc A862 (204.5, 85) -> (200.1, 85) centre (202.3, 85) ccw construction
  line L191 (204.5, 85) -> (204.5, 65) construction
  arc A863 (200.1, 65) -> (204.5, 65) centre (202.3, 65) ccw construction
  line L192 (200.1, 65) -> (200.1, 85) construction
  arc A864 (204.5, 128.5) -> (200.1, 128.5) centre (202.3, 128.5) ccw construction
  line L193 (204.5, 128.5) -> (204.5, 108.5) construction
  arc A865 (200.1, 108.5) -> (204.5, 108.5) centre (202.3, 108.5) ccw construction
  line L194 (200.1, 108.5) -> (200.1, 128.5) construction
  arc A866 (135, 200.1) -> (135, 204.5) centre (135, 202.3) ccw construction
  line L195 (135, 200.1) -> (115, 200.1) construction
  arc A867 (115, 204.5) -> (115, 200.1) centre (115, 202.3) ccw construction
  line L196 (115, 204.5) -> (135, 204.5) construction
  arc A868 (85, 200.1) -> (85, 204.5) centre (85, 202.3) ccw construction
  line L197 (85, 200.1) -> (65, 200.1) construction
  arc A869 (65, 204.5) -> (65, 200.1) centre (65, 202.3) ccw construction
  line L198 (65, 204.5) -> (85, 204.5) construction
  arc A870 (35, 200.1) -> (35, 204.5) centre (35, 202.3) ccw construction
  line L199 (35, 200.1) -> (15, 200.1) construction
  arc A871 (15, 204.5) -> (15, 200.1) centre (15, 202.3) ccw construction
  line L200 (15, 204.5) -> (35, 204.5) construction
  arc A872 (-15, 200.1) -> (-15, 204.5) centre (-15, 202.3) ccw construction
  line L201 (-15, 200.1) -> (-35, 200.1) construction
  arc A873 (-35, 204.5) -> (-35, 200.1) centre (-35, 202.3) ccw construction
  line L202 (-35, 204.5) -> (-15, 204.5) construction
  arc A874 (-65, 200.1) -> (-65, 204.5) centre (-65, 202.3) ccw construction
  line L203 (-65, 200.1) -> (-85, 200.1) construction
  arc A875 (-85, 204.5) -> (-85, 200.1) centre (-85, 202.3) ccw construction
  line L204 (-85, 204.5) -> (-65, 204.5) construction
  arc A876 (-200.1, 128.5) -> (-204.5, 128.5) centre (-202.3, 128.5) ccw construction
  line L205 (-200.1, 128.5) -> (-200.1, 108.5) construction
  arc A877 (-204.5, 108.5) -> (-200.1, 108.5) centre (-202.3, 108.5) ccw construction
  line L206 (-204.5, 108.5) -> (-204.5, 128.5) construction
  arc A878 (-200.1, 85) -> (-204.5, 85) centre (-202.3, 85) ccw construction
  line L207 (-200.1, 85) -> (-200.1, 65) construction
  arc A879 (-204.5, 65) -> (-200.1, 65) centre (-202.3, 65) ccw construction
  line L208 (-204.5, 65) -> (-204.5, 85) construction
  arc A880 (-200.1, 35) -> (-204.5, 35) centre (-202.3, 35) ccw construction
  line L209 (-200.1, 35) -> (-200.1, 15) construction
  arc A881 (-204.5, 15) -> (-200.1, 15) centre (-202.3, 15) ccw construction
  line L210 (-204.5, 15) -> (-204.5, 35) construction
  arc A882 (-200.1, -15) -> (-204.5, -15) centre (-202.3, -15) ccw construction
  line L211 (-200.1, -15) -> (-200.1, -35) construction
  arc A883 (-204.5, -35) -> (-200.1, -35) centre (-202.3, -35) ccw construction
  line L212 (-204.5, -35) -> (-204.5, -15) construction
  arc A884 (-200.1, -65) -> (-204.5, -65) centre (-202.3, -65) ccw construction
  line L213 (-200.1, -65) -> (-200.1, -85) construction
  arc A885 (-204.5, -85) -> (-200.1, -85) centre (-202.3, -85) ccw construction
  line L214 (-204.5, -85) -> (-204.5, -65) construction
  arc A886 (-200.1, -108.5) -> (-204.5, -108.5) centre (-202.3, -108.5) ccw construction
  line L215 (-200.1, -108.5) -> (-200.1, -128.5) construction
  arc A887 (-204.5, -128.5) -> (-200.1, -128.5) centre (-202.3, -128.5) ccw construction
  line L216 (-204.5, -128.5) -> (-204.5, -108.5) construction
  arc A888 (-115, -204.5) -> (-115, -200.1) centre (-115, -202.3) ccw construction
  line L217 (-115, -204.5) -> (-135, -204.5) construction
  arc A889 (-135, -200.1) -> (-135, -204.5) centre (-135, -202.3) ccw construction
  line L218 (-135, -200.1) -> (-115, -200.1) construction
  arc A890 (-65, -204.5) -> (-65, -200.1) centre (-65, -202.3) ccw construction
  line L219 (-65, -204.5) -> (-85, -204.5) construction
  arc A891 (-85, -200.1) -> (-85, -204.5) centre (-85, -202.3) ccw construction
  line L220 (-85, -200.1) -> (-65, -200.1) construction
  arc A892 (85, -204.5) -> (85, -200.1) centre (85, -202.3) ccw construction
  line L221 (85, -204.5) -> (65, -204.5) construction
  arc A893 (65, -200.1) -> (65, -204.5) centre (65, -202.3) ccw construction
  line L222 (65, -200.1) -> (85, -200.1) construction
  arc A894 (135, -204.5) -> (135, -200.1) centre (135, -202.3) ccw construction
  line L223 (135, -204.5) -> (115, -204.5) construction
  arc A895 (115, -200.1) -> (115, -204.5) centre (115, -202.3) ccw construction
  line L224 (115, -200.1) -> (135, -200.1) construction
  arc A896 (159.9476, 195.3029) -> (156.1292, 191.4845) centre (158.0384, 193.3937) ccw construction
  line L225 (159.9476, 195.3029) -> (195.3029, 159.9476) construction
  arc A897 (191.4845, 156.1292) -> (195.3029, 159.9476) centre (193.3937, 158.0384) ccw construction
  line L226 (191.4845, 156.1292) -> (156.1292, 191.4845) construction
  arc A898 (-191.4845, -156.1292) -> (-195.3029, -159.9476) centre (-193.3937, -158.0384) ccw construction
  line L227 (-191.4845, -156.1292) -> (-156.1292, -191.4845) construction
  arc A899 (-159.9476, -195.3029) -> (-156.1292, -191.4845) centre (-158.0384, -193.3937) ccw construction
  line L228 (-159.9476, -195.3029) -> (-195.3029, -159.9476) construction
  circle A900 centre (50, -50) radius 2.15
  circle A901 centre (0, -50) radius 2.15
  circle A902 centre (-50, -50) radius 2.15
  circle A903 centre (50, 0) radius 2.15
  circle A904 centre (50, 50) radius 2.15
  circle A905 centre (-50, 50) radius 2.15
  circle A906 centre (0, 50) radius 2.15
  circle A907 centre (-44.1521, -25.3532) radius 4.48
  circle A908 centre (-50, 0) radius 2.15
  circle A909 centre (-25.3532, 44.1521) radius 4.48
  circle A910 centre (44.1521, 25.3532) radius 4.48
  circle A911 centre (25.3532, -44.1521) radius 4.48
  circle A912 centre (0, 0) radius 16.7
  circle A913 centre (0, 0) radius 42.6559
  circle A914 centre (-50, 0) radius 8.8748
  circle A915 centre (-50, 50) radius 16.1064
  point P0 (5.0637, 57.15)
  point P1 (-5.0637, 57.15)
  point P2 (-44.9363, 57.15)
  point P3 (-55.0637, 57.15)
  point P4 (-57.15, 55.0637)
  point P5 (-57.15, 44.9363)
  point P6 (-57.15, 5.0637)
  point P7 (-57.15, -5.0637)
  point P8 (-57.15, -44.9363)
  point P9 (-57.15, -55.0637)
  point P10 (-55.0637, -57.15)
  point P11 (-44.9363, -57.15)
  point P12 (-5.0637, -57.15)
  point P13 (5.0637, -57.15)
  point P14 (44.9363, -57.15)
  point P15 (55.0637, -57.15)
  point P16 (57.15, -55.0637)
  point P17 (57.15, -44.9363)
  point P18 (57.15, -5.0637)
  point P19 (57.15, 5.0637)
  point P20 (57.15, 44.9363)
  point P21 (57.15, 55.0637)
  point P22 (55.0637, 57.15)
  point P23 (44.9363, 57.15)
  point P24 (-21.9023, 36.6035)
  point P25 (-20.2989, 37.5164)
  point P26 (-19.7407, 37.8132)
  point P27 (5.1229, 42.3472)
  point P28 (36.6035, 21.9023)
  point P29 (37.5164, 20.2989)
  point P30 (37.8132, 19.7407)
  point P31 (42.3472, -5.1229)
  point P32 (21.9023, -36.6035)
  point P33 (20.2989, -37.5164)
  point P34 (19.7407, -37.8132)
  point P35 (-5.1229, -42.3472)
  point P36 (-36.6035, -21.9023)
  point P37 (-37.5164, -20.2989)
  point P38 (-37.8132, -19.7407)
  point P39 (-42.3472, 5.1229)
  dimension "d0" = 114.3
  dimension "d1" = 114.3
  dimension "d4" = 85.3119
  constraints: 16 centre point, 16 coincident, 13 concentric, 12 end point, 3 horizontal, 2 parallel, 2 tangent, 2 vertical, 1 perpendicular, 2 other
  measures "d0" distance of L0.start L0.end
  measures "d1" distance of L0.end L1.end
  measures "d4" diameter of A913
extrude "Extrusion1" add sketch "Sketch1" along normal blind 3.175 contours L0 A671 A670 A669 A663 A662 A661 A548 L1 A542 A541 A540 A914 A913 A533 A532 A531 A530 A537 A585 A584 A583 A582 A581 A573 A572 A571 A570 A577 A525 A524 A523 A915 A402 A401 L2 A348 A347 A346 A340 L3 A586 A593 A592 A594 A601 A600 A677 | L1 A518 A914 A913 A540 | A518 A517 A915 A523 A522 A529 A914 | A914 A529 A913 | A403 A402 A915 A517 A516 L1 A409 L2
sketch "Sketch2" plane through (0, 0, 0) normal (0, 0, -1) x (-1, 0, 0)
  circle A0 centre (0, 0) radius 52.7685
  circle A1 centre (0, 0) radius 55.9435
  dimension "d5" = 105.537
  dimension "d6" = 3.175
  constraints: 2 centre point, 2 coincident
  measures "d5" diameter of A0
  measures "d6" radial gap between concentric circles of A0 A1
extrude "Extrusion3" add sketch "Sketch2" along normal blind 38.1 and the other way blind 3.175
sketch "Sketch4" plane through (0, 0, -38.1) normal (0, 0, -1) x (-1, 0, 0)
  circle A0 centre (-50, 50) radius 2.15 projected
  circle A1 centre (50, -50) radius 2.15 projected
  line L0 (-50, 50) -> (50, 50)
  line L1 (50, 50) -> (50, -50)
  line L2 (50, -50) -> (-50, -50)
  line L3 (-50, -50) -> (-50, 50)
  point P0 (0, 0)
  point P1 (-50, 47.85)
  point P2 (47.85, -50)
  point P3 (50, -47.85)
  point P4 (-47.85, 50)
  constraints: 8 end point, 2 parallel, 1 horizontal, 1 perpendicular
extrude "Extrusion4" cut sketch "Sketch4" against normal up to surface (38.1 mm away) contours L0 L1 A1 L2 L3 A0
sketch "Sketch5" plane through (-5.0637, -57.15, 0) normal (0, -1, 0) x (1, 0, 0)
  line L0 (0, 0) -> (10.1273, 0) projected
  line L1 (10.1273, 0) -> (10.1273, 3.175) projected
  line L2 (0, 3.175) -> (10.1273, 3.175) projected
  line L3 (0, 0) -> (0, 3.175) projected
  line L4 (17.7637, -31.75) -> (-7.6363, -31.75)
  line L5 (-7.6363, -31.75) -> (-7.6363, -25.4)
  line L6 (-7.6363, -25.4) -> (17.7637, -25.4)
  line L7 (17.7637, -25.4) -> (17.7637, -31.75)
  line L8 (5.0637, 3.175) -> (5.0637, 0) construction
  line L9 (-20.0297, -38.1) -> (30.157, -38.1) construction
  dimension "d15" = 25.4
  dimension "d16" = 6.35
  dimension "d17" = 6.35
  constraints: 10 end point, 2 parallel, 1 horizontal, 1 midpoint, 1 perpendicular, 1 vertical, 1 other
  measures "d15" distance of L4.start L4.end
  measures "d16" distance of L4.end L5.end
  measures "d17" distance between parallel lines of L9 L4
extrude "Extrusion5" add sketch "Sketch5" against normal up to surface contours L4 L5 L6 L7 round surface about axis through (0, 0, 0) along (0, 0, -1) radius 52.7685 far side no
extrude "Extrusion6" add sketch "Sketch5" along normal blind 6.35 contours L4 L5 L6 L7